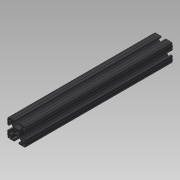
# Autodesk Inventor part: 1515-UL
Saved by Autodesk Inventor 2013 (Build 170138000, 138)
## iProperties
Company: 80/20 Inc.
Created: 2014-04-23
Part Number: 1515-UL
Material: Generic
Document SubType Name: Modeling
Density: 1 g/cm^3
Vendor: 80/20 Inc.
Engineer: Ross Bowman
Designer: Ross Bowman
Catalog Web Link: 8020.net
Material: 6105-T5 Aluminum
Author: Ross Bowman
Keywords: 80/20 , 8020 , T-Slot , Extrusion
Autodesk Inventor part; units mm, degrees
ref_plane "YZ Plane" through (0, 0, 0) normal (1, 0, 0) x (0, 1, 0)
ref_plane "XZ Plane" through (0, 0, 0) normal (0, 1, 0) x (-1, 0, 0)
ref_plane "XY Plane" through (0, 0, 0) normal (0, 0, 1) x (1, 0, 0)
sketch "Sketch1" plane through (0, 0, 0) normal (0, 0, 1) x (1, 0, 0)
  arc A0 (14.0194, 11.8669) -> (14.0212, 11.8676) centre (14.0194, 11.8694) ccw
  line L0 (12.2479, 11.8669) -> (14.0194, 11.8669)
  arc A1 (11.8669, 12.2479) -> (12.2479, 11.8669) centre (12.2479, 12.2479) ccw
  line L1 (11.8669, 14.0195) -> (11.8669, 12.2479)
  arc A2 (11.8676, 14.0213) -> (11.8669, 14.0195) centre (11.8694, 14.0195) ccw
  line L2 (12.4039, 14.5575) -> (11.8676, 14.0213)
  arc A3 (12.4039, 14.5575) -> (12.4039, 14.5611) centre (12.4021, 14.5593) ccw
  line L3 (11.8676, 15.0973) -> (12.4039, 14.5611)
  arc A4 (11.8669, 15.0991) -> (11.8676, 15.0973) centre (11.8694, 15.0991) ccw
  line L4 (11.8669, 16.8707) -> (11.8669, 15.0991)
  arc A5 (12.2479, 17.2517) -> (11.8669, 16.8707) centre (12.2479, 16.8707) ccw
  line L5 (14.4577, 17.2517) -> (12.2479, 17.2517)
  arc A6 (17.2517, 14.4577) -> (14.4577, 17.2517) centre (14.4577, 14.4577) ccw
  line L6 (17.2517, 12.2479) -> (17.2517, 14.4577)
  arc A7 (16.8707, 11.8669) -> (17.2517, 12.2479) centre (16.8707, 12.2479) ccw
  line L7 (15.0991, 11.8669) -> (16.8707, 11.8669)
  arc A8 (15.0973, 11.8676) -> (15.0991, 11.8669) centre (15.0991, 11.8694) ccw
  line L8 (14.5611, 12.4039) -> (15.0973, 11.8676)
  arc A9 (14.5611, 12.4039) -> (14.5575, 12.4039) centre (14.5593, 12.4021) ccw
  line L9 (14.0212, 11.8676) -> (14.5575, 12.4039)
  arc A10 (11.8669, -14.0194) -> (11.8676, -14.0212) centre (11.8694, -14.0194) ccw
  line L10 (11.8669, -12.2479) -> (11.8669, -14.0194)
  arc A11 (12.2479, -11.8669) -> (11.8669, -12.2479) centre (12.2479, -12.2479) ccw
  line L11 (14.0195, -11.8669) -> (12.2479, -11.8669)
  arc A12 (14.0213, -11.8676) -> (14.0195, -11.8669) centre (14.0195, -11.8694) ccw
  line L12 (14.5575, -12.4039) -> (14.0213, -11.8676)
  arc A13 (14.5575, -12.4039) -> (14.5611, -12.4039) centre (14.5593, -12.4021) ccw
  line L13 (15.0973, -11.8676) -> (14.5611, -12.4039)
  arc A14 (15.0991, -11.8669) -> (15.0973, -11.8676) centre (15.0991, -11.8694) ccw
  line L14 (16.8707, -11.8669) -> (15.0991, -11.8669)
  arc A15 (17.2517, -12.2479) -> (16.8707, -11.8669) centre (16.8707, -12.2479) ccw
  line L15 (17.2517, -14.4577) -> (17.2517, -12.2479)
  arc A16 (14.4577, -17.2517) -> (17.2517, -14.4577) centre (14.4577, -14.4577) ccw
  line L16 (12.2479, -17.2517) -> (14.4577, -17.2517)
  arc A17 (11.8669, -16.8707) -> (12.2479, -17.2517) centre (12.2479, -16.8707) ccw
  line L17 (11.8669, -15.0991) -> (11.8669, -16.8707)
  arc A18 (11.8676, -15.0973) -> (11.8669, -15.0991) centre (11.8694, -15.0991) ccw
  line L18 (12.4039, -14.5611) -> (11.8676, -15.0973)
  arc A19 (12.4039, -14.5611) -> (12.4039, -14.5575) centre (12.4021, -14.5593) ccw
  line L19 (11.8676, -14.0212) -> (12.4039, -14.5575)
  arc A20 (-14.0194, -11.8669) -> (-14.0212, -11.8676) centre (-14.0194, -11.8694) ccw
  line L20 (-12.2479, -11.8669) -> (-14.0194, -11.8669)
  arc A21 (-11.8669, -12.2479) -> (-12.2479, -11.8669) centre (-12.2479, -12.2479) ccw
  line L21 (-11.8669, -14.0195) -> (-11.8669, -12.2479)
  arc A22 (-11.8676, -14.0213) -> (-11.8669, -14.0195) centre (-11.8694, -14.0195) ccw
  line L22 (-12.4039, -14.5575) -> (-11.8676, -14.0213)
  arc A23 (-12.4039, -14.5575) -> (-12.4039, -14.5611) centre (-12.4021, -14.5593) ccw
  line L23 (-11.8676, -15.0973) -> (-12.4039, -14.5611)
  arc A24 (-11.8669, -15.0991) -> (-11.8676, -15.0973) centre (-11.8694, -15.0991) ccw
  line L24 (-11.8669, -16.8707) -> (-11.8669, -15.0991)
  arc A25 (-12.2479, -17.2517) -> (-11.8669, -16.8707) centre (-12.2479, -16.8707) ccw
  line L25 (-14.4577, -17.2517) -> (-12.2479, -17.2517)
  arc A26 (-17.2517, -14.4577) -> (-14.4577, -17.2517) centre (-14.4577, -14.4577) ccw
  line L26 (-17.2517, -12.2479) -> (-17.2517, -14.4577)
  arc A27 (-16.8707, -11.8669) -> (-17.2517, -12.2479) centre (-16.8707, -12.2479) ccw
  line L27 (-15.0991, -11.8669) -> (-16.8707, -11.8669)
  arc A28 (-15.0973, -11.8676) -> (-15.0991, -11.8669) centre (-15.0991, -11.8694) ccw
  line L28 (-14.5611, -12.4039) -> (-15.0973, -11.8676)
  arc A29 (-14.5611, -12.4039) -> (-14.5575, -12.4039) centre (-14.5593, -12.4021) ccw
  line L29 (-14.0212, -11.8676) -> (-14.5575, -12.4039)
  arc A30 (-11.8669, 14.0194) -> (-11.8676, 14.0212) centre (-11.8694, 14.0194) ccw
  line L30 (-11.8669, 12.2479) -> (-11.8669, 14.0194)
  arc A31 (-12.2479, 11.8669) -> (-11.8669, 12.2479) centre (-12.2479, 12.2479) ccw
  line L31 (-14.0195, 11.8669) -> (-12.2479, 11.8669)
  arc A32 (-14.0213, 11.8676) -> (-14.0195, 11.8669) centre (-14.0195, 11.8694) ccw
  line L32 (-14.5575, 12.4039) -> (-14.0213, 11.8676)
  arc A33 (-14.5575, 12.4039) -> (-14.5611, 12.4039) centre (-14.5593, 12.4021) ccw
  line L33 (-15.0973, 11.8676) -> (-14.5611, 12.4039)
  arc A34 (-15.0991, 11.8669) -> (-15.0973, 11.8676) centre (-15.0991, 11.8694) ccw
  line L34 (-16.8707, 11.8669) -> (-15.0991, 11.8669)
  arc A35 (-17.2517, 12.2479) -> (-16.8707, 11.8669) centre (-16.8707, 12.2479) ccw
  line L35 (-17.2517, 14.4577) -> (-17.2517, 12.2479)
  arc A36 (-14.4577, 17.2517) -> (-17.2517, 14.4577) centre (-14.4577, 14.4577) ccw
  line L36 (-12.2479, 17.2517) -> (-14.4577, 17.2517)
  arc A37 (-11.8669, 16.8707) -> (-12.2479, 17.2517) centre (-12.2479, 16.8707) ccw
  line L37 (-11.8669, 15.0991) -> (-11.8669, 16.8707)
  arc A38 (-11.8676, 15.0973) -> (-11.8669, 15.0991) centre (-11.8694, 15.0991) ccw
  line L38 (-12.4039, 14.5611) -> (-11.8676, 15.0973)
  arc A39 (-12.4039, 14.5611) -> (-12.4039, 14.5575) centre (-12.4021, 14.5593) ccw
  line L39 (-11.8676, 14.0212) -> (-12.4039, 14.5575)
  arc A40 (1.178, 3.1119) -> (-1.178, 3.1119) centre (0, 0) ccw
  arc A41 (1.178, 3.1119) -> (1.5823, 3.1988) centre (1.3129, 3.4682) ccw
  line L40 (3.2921, 4.9085) -> (1.5823, 3.1988)
  arc A42 (3.9207, 5.1689) -> (3.2921, 4.9085) centre (3.9207, 4.2799) ccw
  line L41 (4.9149, 5.1689) -> (3.9207, 5.1689)
  arc A43 (5.1689, 4.9149) -> (4.9149, 5.1689) centre (4.9149, 4.9149) ccw
  line L42 (5.1689, 3.9207) -> (5.1689, 4.9149)
  arc A44 (4.9085, 3.2921) -> (5.1689, 3.9207) centre (4.2799, 3.9207) ccw
  line L43 (3.1988, 1.5823) -> (4.9085, 3.2921)
  arc A45 (3.1988, 1.5823) -> (3.1119, 1.178) centre (3.4682, 1.3129) ccw
  arc A46 (3.1119, -1.178) -> (3.1119, 1.178) centre (0, 0) ccw
  arc A47 (3.1119, -1.178) -> (3.1988, -1.5823) centre (3.4682, -1.3129) ccw
  line L44 (4.9085, -3.2921) -> (3.1988, -1.5823)
  arc A48 (5.1689, -3.9207) -> (4.9085, -3.2921) centre (4.2799, -3.9207) ccw
  line L45 (5.1689, -4.9149) -> (5.1689, -3.9207)
  arc A49 (4.9149, -5.1689) -> (5.1689, -4.9149) centre (4.9149, -4.9149) ccw
  line L46 (3.9207, -5.1689) -> (4.9149, -5.1689)
  arc A50 (3.2921, -4.9085) -> (3.9207, -5.1689) centre (3.9207, -4.2799) ccw
  line L47 (1.5823, -3.1988) -> (3.2921, -4.9085)
  arc A51 (1.5823, -3.1988) -> (1.178, -3.1119) centre (1.3129, -3.4682) ccw
  arc A52 (-1.178, -3.1119) -> (1.178, -3.1119) centre (0, 0) ccw
  arc A53 (-1.178, -3.1119) -> (-1.5823, -3.1988) centre (-1.3129, -3.4682) ccw
  line L48 (-3.2921, -4.9085) -> (-1.5823, -3.1988)
  arc A54 (-3.9207, -5.1689) -> (-3.2921, -4.9085) centre (-3.9207, -4.2799) ccw
  line L49 (-4.9149, -5.1689) -> (-3.9207, -5.1689)
  arc A55 (-5.1689, -4.9149) -> (-4.9149, -5.1689) centre (-4.9149, -4.9149) ccw
  line L50 (-5.1689, -3.9207) -> (-5.1689, -4.9149)
  arc A56 (-4.9085, -3.2921) -> (-5.1689, -3.9207) centre (-4.2799, -3.9207) ccw
  line L51 (-3.1988, -1.5823) -> (-4.9085, -3.2921)
  arc A57 (-3.1988, -1.5823) -> (-3.1119, -1.178) centre (-3.4682, -1.3129) ccw
  arc A58 (-3.1119, 1.178) -> (-3.1119, -1.178) centre (0, 0) ccw
  arc A59 (-3.1119, 1.178) -> (-3.1988, 1.5823) centre (-3.4682, 1.3129) ccw
  line L52 (-4.9085, 3.2921) -> (-3.1988, 1.5823)
  arc A60 (-5.1689, 3.9207) -> (-4.9085, 3.2921) centre (-4.2799, 3.9207) ccw
  line L53 (-5.1689, 4.9149) -> (-5.1689, 3.9207)
  arc A61 (-4.9149, 5.1689) -> (-5.1689, 4.9149) centre (-4.9149, 4.9149) ccw
  line L54 (-3.9207, 5.1689) -> (-4.9149, 5.1689)
  arc A62 (-3.2921, 4.9085) -> (-3.9207, 5.1689) centre (-3.9207, 4.2799) ccw
  line L55 (-1.5823, 3.1988) -> (-3.2921, 4.9085)
  arc A63 (-1.5823, 3.1988) -> (-1.178, 3.1119) centre (-1.3129, 3.4682) ccw
  arc A64 (6.731, -15.3661) -> (6.3498, -14.9848) centre (6.35, -15.3658) ccw
  line L56 (6.3498, -14.9848) -> (5.6531, -14.9848)
  arc A65 (5.6531, -14.9848) -> (4.0778, -16.5601) centre (5.6526, -16.5596) ccw
  line L57 (4.0778, -16.5601) -> (4.0778, -17.4747)
  arc A66 (4.0778, -17.4747) -> (5.6531, -19.05) centre (5.6526, -17.4752) ccw
  line L58 (5.6531, -19.05) -> (7.9756, -19.05)
  arc A67 (9.4996, -19.05) -> (7.9756, -19.05) centre (8.7376, -19.05) ccw
  line L59 (9.4996, -19.05) -> (14.2981, -19.05)
  arc A68 (15.8221, -19.0496) -> (14.2981, -19.05) centre (15.0601, -19.05) ccw
  arc A69 (15.8221, -19.0496) -> (19.0499, -15.8496) centre (15.875, -15.875) ccw
  arc A70 (19.05, -14.3256) -> (19.0499, -15.8496) centre (19.05, -15.0876) ccw
  line L60 (19.05, -14.3256) -> (19.05, -9.4996)
  arc A71 (19.05, -7.9756) -> (19.05, -9.4996) centre (19.05, -8.7376) ccw
  line L61 (19.05, -7.9756) -> (19.05, -5.6531)
  arc A72 (19.05, -5.6531) -> (17.4747, -4.0778) centre (17.4752, -5.6526) ccw
  line L62 (17.4747, -4.0778) -> (16.5601, -4.0778)
  arc A73 (16.5601, -4.0778) -> (14.9848, -5.6531) centre (16.5596, -5.6526) ccw
  line L63 (14.9848, -5.6531) -> (14.9848, -6.3498)
  arc A74 (14.9848, -6.3498) -> (15.3661, -6.731) centre (15.3658, -6.35) ccw
  line L64 (15.3661, -6.731) -> (15.6969, -6.731)
  arc A75 (16.0782, -7.1122) -> (15.6969, -6.731) centre (15.6972, -7.112) ccw
  line L65 (16.0782, -7.1122) -> (16.0782, -9.3968)
  arc A76 (15.1881, -10.287) -> (16.0782, -9.3968) centre (15.1892, -9.398) ccw
  line L66 (15.1881, -10.287) -> (12.3526, -10.2871)
  arc A77 (11.4535, -9.9142) -> (12.3526, -10.2871) centre (12.3525, -9.0171) ccw
  line L67 (11.4535, -9.9142) -> (7.1147, -5.5659)
  arc A78 (6.7437, -4.6689) -> (7.1147, -5.5659) centre (8.0137, -4.6689) ccw
  line L68 (6.7437, -4.6689) -> (6.7437, 4.6414)
  arc A79 (7.1147, 5.5384) -> (6.7437, 4.6414) centre (8.0137, 4.6414) ccw
  line L69 (7.1147, 5.5384) -> (11.481, 9.9142)
  arc A80 (12.38, 10.2871) -> (11.481, 9.9142) centre (12.38, 9.0171) ccw
  line L70 (12.38, 10.2871) -> (15.1881, 10.287)
  arc A81 (16.0782, 9.3968) -> (15.1881, 10.287) centre (15.1892, 9.398) ccw
  line L71 (16.0782, 9.3968) -> (16.0782, 7.1122)
  arc A82 (15.6969, 6.731) -> (16.0782, 7.1122) centre (15.6972, 7.112) ccw
  line L72 (15.6969, 6.731) -> (15.3661, 6.731)
  arc A83 (15.3661, 6.731) -> (14.9848, 6.3498) centre (15.3658, 6.35) ccw
  line L73 (14.9848, 6.3498) -> (14.9848, 5.6531)
  arc A84 (14.9848, 5.6531) -> (16.5601, 4.0778) centre (16.5596, 5.6526) ccw
  line L74 (16.5601, 4.0778) -> (17.4747, 4.0778)
  arc A85 (17.4747, 4.0778) -> (19.05, 5.6531) centre (17.4752, 5.6526) ccw
  line L75 (19.05, 5.6531) -> (19.05, 7.9756)
  arc A86 (19.05, 9.4996) -> (19.05, 7.9756) centre (19.05, 8.7376) ccw
  line L76 (19.05, 9.4996) -> (19.05, 14.2981)
  arc A87 (19.0496, 15.8221) -> (19.05, 14.2981) centre (19.05, 15.0601) ccw
  arc A88 (19.0496, 15.8221) -> (15.8496, 19.0499) centre (15.875, 15.875) ccw
  arc A89 (14.3256, 19.05) -> (15.8496, 19.0499) centre (15.0876, 19.05) ccw
  line L77 (14.3256, 19.05) -> (9.4996, 19.05)
  arc A90 (7.9756, 19.05) -> (9.4996, 19.05) centre (8.7376, 19.05) ccw
  line L78 (7.9756, 19.05) -> (5.6531, 19.05)
  arc A91 (5.6531, 19.05) -> (4.0778, 17.4747) centre (5.6526, 17.4752) ccw
  line L79 (4.0778, 17.4747) -> (4.0778, 16.5601)
  arc A92 (4.0778, 16.5601) -> (5.6531, 14.9848) centre (5.6526, 16.5596) ccw
  line L80 (5.6531, 14.9848) -> (6.3498, 14.9848)
  arc A93 (6.3498, 14.9848) -> (6.731, 15.3661) centre (6.35, 15.3658) ccw
  line L81 (6.731, 15.3661) -> (6.731, 15.6969)
  arc A94 (7.1122, 16.0782) -> (6.731, 15.6969) centre (7.112, 15.6972) ccw
  line L82 (7.1122, 16.0782) -> (9.3968, 16.0782)
  arc A95 (10.287, 15.1881) -> (9.3968, 16.0782) centre (9.398, 15.1892) ccw
  line L83 (10.287, 15.1881) -> (10.2871, 12.3526)
  arc A96 (9.9142, 11.4535) -> (10.2871, 12.3526) centre (9.0171, 12.3525) ccw
  line L84 (9.9142, 11.4535) -> (5.5659, 7.1147)
  arc A97 (4.6689, 6.7437) -> (5.5659, 7.1147) centre (4.6689, 8.0137) ccw
  line L85 (4.6689, 6.7437) -> (-4.6414, 6.7437)
  arc A98 (-5.5384, 7.1147) -> (-4.6414, 6.7437) centre (-4.6414, 8.0137) ccw
  line L86 (-5.5384, 7.1147) -> (-9.9142, 11.481)
  arc A99 (-10.2871, 12.38) -> (-9.9142, 11.481) centre (-9.0171, 12.38) ccw
  line L87 (-10.2871, 12.38) -> (-10.287, 15.1881)
  arc A100 (-9.3968, 16.0782) -> (-10.287, 15.1881) centre (-9.398, 15.1892) ccw
  line L88 (-9.3968, 16.0782) -> (-7.1122, 16.0782)
  arc A101 (-6.731, 15.6969) -> (-7.1122, 16.0782) centre (-7.112, 15.6972) ccw
  line L89 (-6.731, 15.6969) -> (-6.731, 15.3661)
  arc A102 (-6.731, 15.3661) -> (-6.3498, 14.9848) centre (-6.35, 15.3658) ccw
  line L90 (-6.3498, 14.9848) -> (-5.6531, 14.9848)
  arc A103 (-5.6531, 14.9848) -> (-4.0778, 16.5601) centre (-5.6526, 16.5596) ccw
  line L91 (-4.0778, 16.5601) -> (-4.0778, 17.4747)
  arc A104 (-4.0778, 17.4747) -> (-5.6531, 19.05) centre (-5.6526, 17.4752) ccw
  line L92 (-5.6531, 19.05) -> (-7.9756, 19.05)
  arc A105 (-9.4996, 19.05) -> (-7.9756, 19.05) centre (-8.7376, 19.05) ccw
  line L93 (-9.4996, 19.05) -> (-14.2981, 19.05)
  arc A106 (-15.8221, 19.0496) -> (-14.2981, 19.05) centre (-15.0601, 19.05) ccw
  arc A107 (-15.8221, 19.0496) -> (-19.0499, 15.8496) centre (-15.875, 15.875) ccw
  arc A108 (-19.05, 14.3256) -> (-19.0499, 15.8496) centre (-19.05, 15.0876) ccw
  line L94 (-19.05, 14.3256) -> (-19.05, 9.4996)
  arc A109 (-19.05, 7.9756) -> (-19.05, 9.4996) centre (-19.05, 8.7376) ccw
  line L95 (-19.05, 7.9756) -> (-19.05, 5.6531)
  arc A110 (-19.05, 5.6531) -> (-17.4747, 4.0778) centre (-17.4752, 5.6526) ccw
  line L96 (-17.4747, 4.0778) -> (-16.5601, 4.0778)
  arc A111 (-16.5601, 4.0778) -> (-14.9848, 5.6531) centre (-16.5596, 5.6526) ccw
  line L97 (-14.9848, 5.6531) -> (-14.9848, 6.3498)
  arc A112 (-14.9848, 6.3498) -> (-15.3661, 6.731) centre (-15.3658, 6.35) ccw
  line L98 (-15.3661, 6.731) -> (-15.6969, 6.731)
  arc A113 (-16.0782, 7.1122) -> (-15.6969, 6.731) centre (-15.6972, 7.112) ccw
  line L99 (-16.0782, 7.1122) -> (-16.0782, 9.3968)
  arc A114 (-15.1881, 10.287) -> (-16.0782, 9.3968) centre (-15.1892, 9.398) ccw
  line L100 (-15.1881, 10.287) -> (-12.3526, 10.2871)
  arc A115 (-11.4535, 9.9142) -> (-12.3526, 10.2871) centre (-12.3525, 9.0171) ccw
  line L101 (-11.4535, 9.9142) -> (-7.1147, 5.5659)
  arc A116 (-6.7437, 4.6689) -> (-7.1147, 5.5659) centre (-8.0137, 4.6689) ccw
  line L102 (-6.7437, 4.6689) -> (-6.7437, -4.6414)
  arc A117 (-7.1147, -5.5384) -> (-6.7437, -4.6414) centre (-8.0137, -4.6414) ccw
  line L103 (-7.1147, -5.5384) -> (-11.481, -9.9142)
  arc A118 (-12.38, -10.2871) -> (-11.481, -9.9142) centre (-12.38, -9.0171) ccw
  line L104 (-12.38, -10.2871) -> (-15.1881, -10.287)
  arc A119 (-16.0782, -9.3968) -> (-15.1881, -10.287) centre (-15.1892, -9.398) ccw
  line L105 (-16.0782, -9.3968) -> (-16.0782, -7.1122)
  arc A120 (-15.6969, -6.731) -> (-16.0782, -7.1122) centre (-15.6972, -7.112) ccw
  line L106 (-15.6969, -6.731) -> (-15.3661, -6.731)
  arc A121 (-15.3661, -6.731) -> (-14.9848, -6.3498) centre (-15.3658, -6.35) ccw
  line L107 (-14.9848, -6.3498) -> (-14.9848, -5.6531)
  arc A122 (-14.9848, -5.6531) -> (-16.5601, -4.0778) centre (-16.5596, -5.6526) ccw
  line L108 (-16.5601, -4.0778) -> (-17.4747, -4.0778)
  arc A123 (-17.4747, -4.0778) -> (-19.05, -5.6531) centre (-17.4752, -5.6526) ccw
  line L109 (-19.05, -5.6531) -> (-19.05, -7.9756)
  arc A124 (-19.05, -9.4996) -> (-19.05, -7.9756) centre (-19.05, -8.7376) ccw
  line L110 (-19.05, -9.4996) -> (-19.05, -14.2981)
  arc A125 (-19.0496, -15.8221) -> (-19.05, -14.2981) centre (-19.05, -15.0601) ccw
  arc A126 (-19.0496, -15.8221) -> (-15.8496, -19.0499) centre (-15.875, -15.875) ccw
  arc A127 (-14.3256, -19.05) -> (-15.8496, -19.0499) centre (-15.0876, -19.05) ccw
  line L111 (-14.3256, -19.05) -> (-9.4996, -19.05)
  arc A128 (-7.9756, -19.05) -> (-9.4996, -19.05) centre (-8.7376, -19.05) ccw
  line L112 (-7.9756, -19.05) -> (-5.6531, -19.05)
  arc A129 (-5.6531, -19.05) -> (-4.0778, -17.4747) centre (-5.6526, -17.4752) ccw
  line L113 (-4.0778, -17.4747) -> (-4.0778, -16.5601)
  arc A130 (-4.0778, -16.5601) -> (-5.6531, -14.9848) centre (-5.6526, -16.5596) ccw
  line L114 (-5.6531, -14.9848) -> (-6.3498, -14.9848)
  arc A131 (-6.3498, -14.9848) -> (-6.731, -15.3661) centre (-6.35, -15.3658) ccw
  line L115 (-6.731, -15.3661) -> (-6.731, -15.6969)
  arc A132 (-7.1122, -16.0782) -> (-6.731, -15.6969) centre (-7.112, -15.6972) ccw
  line L116 (-7.1122, -16.0782) -> (-9.3968, -16.0782)
  arc A133 (-10.287, -15.1881) -> (-9.3968, -16.0782) centre (-9.398, -15.1892) ccw
  line L117 (-10.287, -15.1881) -> (-10.2871, -12.3526)
  arc A134 (-9.9142, -11.4535) -> (-10.2871, -12.3526) centre (-9.0171, -12.3525) ccw
  line L118 (-9.9142, -11.4535) -> (-5.5659, -7.1147)
  arc A135 (-4.6689, -6.7437) -> (-5.5659, -7.1147) centre (-4.6689, -8.0137) ccw
  line L119 (-4.6689, -6.7437) -> (4.6414, -6.7437)
  arc A136 (5.5384, -7.1147) -> (4.6414, -6.7437) centre (4.6414, -8.0137) ccw
  line L120 (5.5384, -7.1147) -> (9.9142, -11.481)
  arc A137 (10.2871, -12.38) -> (9.9142, -11.481) centre (9.0171, -12.38) ccw
  line L121 (10.2871, -12.38) -> (10.287, -15.1881)
  arc A138 (9.3968, -16.0782) -> (10.287, -15.1881) centre (9.398, -15.1892) ccw
  line L122 (9.3968, -16.0782) -> (7.1122, -16.0782)
  arc A139 (6.731, -15.6969) -> (7.1122, -16.0782) centre (7.112, -15.6972) ccw
  line L123 (6.731, -15.6969) -> (6.731, -15.3661)
  constraints: 280 point on circle, 248 end point, 140 centre point
extrude "Extrusion1" add sketch "Sketch1" against normal blind 304.8
body "Solid1"
